Autodesk Fusion 360 part; units mm, degrees
(part 2 of 2)
copy_body "Body->Comp1" bodies 1 removing the originals makes body 2 in component "Wheel"
sketch "Sketch3" plane through (0, 0, 0) normal (0, 1, 0) x (1, 0, 0)
  circle A0 centre (0, 0) radius 7
  dimension "d37" = 14
  constraint coincident A0.centre origin
  measures "d37" diameter of A0
extrude "Extrude1'" add sketch "Sketch3" against normal blind 39 bodies 2 in component "Wheel"
sketch "Sketch4" plane through (0, 0, 0) normal (0, 1, 0) x (1, 0, 0)
  line L0 (1.5, -2) -> (1.5, 2)
  line L1 (-1.5, 2) -> (-1.5, -2)
  arc A0 (-1.5, -2) -> (1.5, -2) centre (0, 0) ccw
  arc A1 (1.5, 2) -> (-1.5, 2) centre (0, 0) ccw
  dimension "d40" = 5
  dimension "d41" = 3
  dimension "d42" = 4
  constraint coincident A0.centre A1.centre
  constraint vertical L0
  constraint vertical L1
  constraint concentric A0 A1
  measures "d40" diameter of A0
  measures "d41" distance of L1.end L0.start
  measures "d42" distance of L1.end L1.start
extrude "Extrude2'" cut sketch "Sketch4" along normal blind 6.5 from surface at -39 bodies 2 in component "Wheel"
sketch "Sketch8" plane through (0, 0, 0) normal (0, 1, 0) x (1, 0, 0)
  circle A0 centre (0, 0) radius 4
  dimension "d92" = 8
  constraint coincident A0.centre origin
  measures "d92" diameter of A0
sketch "Sketch9" plane through (0, 0, 0) normal (0, 1, 0) x (1, 0, 0)
  circle A0 centre (0, 0) radius 10
  line L0 (0.6946, -3.9392) -> (1.5628, -8.8633)
  line L1 (4, 0) -> (9, 0) construction
  line L2 (3.9392, -0.6946) -> (8.8633, -1.5628)
  line L3 (4, 0) -> (9, 0) construction
  line L4 (-0.6946, -3.9392) -> (-1.5628, -8.8633)
  line L5 (4, 0) -> (9, 0) construction
  line L6 (-3.9392, -0.6946) -> (-8.8633, -1.5628)
  line L7 (4, 0) -> (9, 0) construction
  line L8 (-3.9392, 0.6946) -> (-8.8633, 1.5628)
  line L9 (4, 0) -> (9, 0) construction
  line L10 (3.9392, 0.6946) -> (8.8633, 1.5628)
  line L11 (4, 0) -> (9, 0) construction
  line L12 (-0.6946, 3.9392) -> (-1.5628, 8.8633)
  line L13 (0.6946, 3.9392) -> (1.5628, 8.8633)
  arc A1 (8.8633, 1.5628) -> (1.5628, 8.8633) centre (0, 0) ccw
  arc A2 (-1.5628, 8.8633) -> (-8.8633, 1.5628) centre (0, 0) ccw
  arc A3 (-8.8633, -1.5628) -> (-1.5628, -8.8633) centre (0, 0) ccw
  arc A4 (1.5628, -8.8633) -> (8.8633, -1.5628) centre (0, 0) ccw
  arc A5 (3.9392, 0.6946) -> (0.6946, 3.9392) centre (0, 0) ccw
  arc A6 (-0.6946, 3.9392) -> (-3.9392, 0.6946) centre (0, 0) ccw
  arc A7 (-3.9392, -0.6946) -> (-0.6946, -3.9392) centre (0, 0) ccw
  arc A8 (0.6946, -3.9392) -> (3.9392, -0.6946) centre (0, 0) ccw
  dimension "d81" = 80
  dimension "d82" = 10
  dimension "d83" = 100
  dimension "d84" = 170
  dimension "d85" = 170
  dimension "d86" = 10
  constraint horizontal L1
  constraint horizontal L3
  constraint horizontal L5
  constraint horizontal L7
  constraint horizontal L9
  constraint horizontal L11
  constraint coincident L12.end A1
  constraint parallel L0 L12
  constraint perpendicular L8 L13
  constraint concentric A1 A2
  constraint concentric A2 A3
  constraint concentric A3 A4
  constraint concentric A1 A5
  constraint coincident L4.start A5
  constraint coincident L6.start A5
  constraint coincident L8.start A5
  constraint coincident L12.start A5
  constraint concentric A5 A6
  constraint concentric A6 A7
  constraint coincident A0.centre A1.centre
  measures "d81" angle of L0 L1
  measures "d82" angle of L2 L3
  measures "d83" angle of L4 L5
  measures "d84" angle of L6 L7
  measures "d85" angle of L8 L9
  measures "d86" angle of L10 L11
extrude "Extrude5" cut sketch "Sketch8" against normal blind 10 from surface at 1 bodies 2 in component "Wheel"
component "Wheel" placed x (1, 0, 0) y (0, 1, 0) z (0, 0, 1) at (0, 0, 0)
